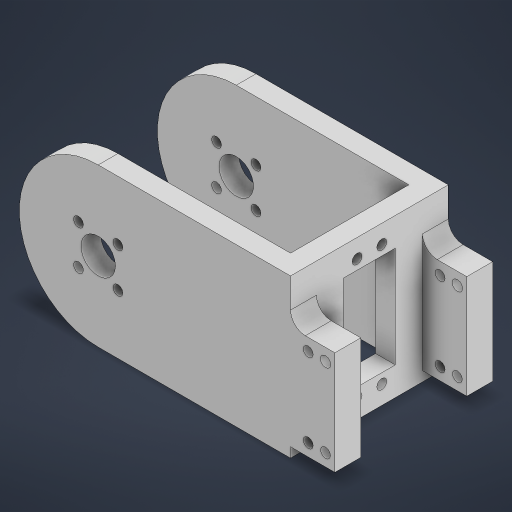
# Autodesk Inventor part: DifferentialMount
Saved by Autodesk Inventor 2024 (Build 280153000, 153)
## iProperties
Created: 2024-01-28
Part Number: DifferentialMount
Material: Generic
Document SubType Name: Modeling
Designer: avsar
Density: 1 g/cm^3
Appearance: Default
Author: avsar
Autodesk Inventor part; units mm, degrees
ref_plane "YZ Plane" through (0, 0, 0) normal (1, 0, 0) x (0, 1, 0)
ref_plane "XZ Plane" through (0, 0, 0) normal (0, 1, 0) x (-1, 0, 0)
ref_plane "XY Plane" through (0, 0, 0) normal (0, 0, 1) x (1, 0, 0)
sketch "Sketch1" plane through (0, 0, 0) normal (1, 0, 0) x (0, 1, 0)
  line L0 (-32, 32) -> (32, 32)
  line L1 (32, 32) -> (32, -32)
  line L2 (32, -32) -> (-32, -32)
  line L3 (-32, -32) -> (-32, 32)
  line L4 (-32, 32) -> (32, -32) construction
  line L5 (32, 32) -> (-32, -32) construction
  point P0 (0, 0)
  dimension "d0" = 64
  dimension "d1" = 64
  constraints: 12 end point, 2 midpoint, 2 parallel, 1 horizontal, 1 perpendicular
  measures "d0" distance of L1.end L2.end
  measures "d1" distance of L0.end L1.end
extrude "Extrusion1" add sketch "Sketch1" along normal blind 8
sketch "Sketch2" plane through (0, 0, 0) normal (-1, 0, 0) x (0, 0, 1)
  line L0 (-32, -32) -> (-24, -32)
  line L1 (-24, -32) -> (-24, 32)
  line L2 (-24, 32) -> (-32, 32)
  line L3 (-32, 32) -> (-32, -32)
  line L4 (-32, -32) -> (-24, 32) construction
  line L5 (-24, -32) -> (-32, 32) construction
  line L6 (-32, -32) -> (-32, 32) projected
  line L7 (-32, 32) -> (32, 32) projected
  line L8 (0, 32) -> (0, -32) construction
  line L9 (32, -32) -> (-32, -32) projected
  line L10 (32, -32) -> (24, -32)
  line L11 (24, -32) -> (24, 32)
  line L12 (24, 32) -> (32, 32)
  line L13 (32, 32) -> (32, -32)
  line L14 (32, -32) -> (24, 32) construction
  line L15 (24, -32) -> (32, 32) construction
  point P0 (0, 0)
  point P1 (-28, 0)
  point P2 (-32, 0)
  point P3 (28, 0)
  point P4 (32, 0)
  dimension "d4" = 8
  dimension "d5" = 64
  constraints: 26 end point, 6 midpoint, 6 symmetric about line, 2 parallel, 1 horizontal, 1 horizontal alignment, 1 perpendicular
  measures "d4" distance of L2.end L1.end
  measures "d5" distance of L1.end L0.end
extrude "Extrusion2" add sketch "Sketch2" along normal blind 102 contours L3 L2 L1 L0 | L11 L7 L13 L9
fillet "Fillet1" radius 32 4 edges at (-102, 32, -28) (-102, 32, 28) (-102, -32, 28) (-102, -32, -28)
sketch "Sketch3" plane through (0, -32, 32) normal (0, 0, 1) x (1, 0, 0)
  arc A0 (-70, 64) -> (-70, 0) centre (-70, 32) ccw construction
  circle A1 centre (-70, 32) radius 7
  circle A2 centre (-78, 40) radius 2
  circle A3 centre (-78, 24) radius 2
  circle A4 centre (-62, 24) radius 2
  circle A5 centre (-62, 40) radius 2
  point P0 (0, 32)
  point P1 (-64, 48)
  dimension "d9" = 14
  dimension "d10" = 4
  dimension "d11" = 8
  dimension "d12" = 8
  dimension "d15" = 360
  constraints: 5 centre point, 1 coincident, 9 other
  measures "d9" diameter of A1
  measures "d10" diameter of A2
  measures "d11" horizontal distance of A2.centre A0.centre
  measures "d12" horizontal distance of A0.centre A2.centre
extrude "Extrusion3" cut sketch "Sketch3" against normal through all
sketch "Sketch5" plane through (8, 0, 0) normal (1, 0, 0) x (0, 0, -1)
  circle A0 centre (-5, 24.5) radius 2
  line L0 (0, 7) -> (0, 0) construction
  circle A1 centre (5, 24.5) radius 2
  circle A2 centre (-5, -24.5) radius 2
  circle A3 centre (5, -24.5) radius 2
  line L1 (-32, 32) -> (-32, -32) construction
  line L2 (-32, 0) -> (32, 0) construction
  line L3 (32, 32) -> (32, -32) construction
  dimension "d22" = 4
  dimension "d23" = 5
  dimension "d24" = 24.5
  constraints: 4 centre point, 4 end point, 2 midpoint, 1 symmetric about line, 1 vertical, 3 other
  measures "d22" diameter of A0
  measures "d23" horizontal distance of point (0, 0) A0.centre
  measures "d24" vertical distance of point (0, 0) A0.centre
extrude "Extrusion5" cut sketch "Sketch5" against normal through all
sketch "Sketch7" plane through (8, 0, 0) normal (1, 0, 0) x (0, 0, -1)
  line L0 (-10.5, -20.5) -> (10.5, -20.5)
  line L1 (10.5, -20.5) -> (10.5, 20.5)
  line L2 (10.5, 20.5) -> (-10.5, 20.5)
  line L3 (-10.5, 20.5) -> (-10.5, -20.5)
  line L4 (-10.5, -20.5) -> (10.5, 20.5) construction
  line L5 (10.5, -20.5) -> (-10.5, 20.5) construction
  point P0 (0, 0)
  dimension "d30" = 21
  dimension "d31" = 41
  constraints: 12 end point, 2 midpoint, 2 parallel, 1 horizontal, 1 perpendicular
  measures "d30" distance of L2.end L1.end
  measures "d31" distance of L1.end L0.end
extrude "Extrusion7" cut sketch "Sketch7" against normal up to surface (8 mm away)
sketch "Sketch8" plane through (8, 0, 0) normal (1, 0, 0) x (0, 0, -1)
  line L0 (-32, -28) -> (-21.5, -28)
  line L1 (-21.5, -28) -> (-21.5, 14)
  line L2 (-21.5, 14) -> (-32, 14)
  line L3 (-32, 14) -> (-32, -28)
  line L4 (-32, -28) -> (-21.5, 14) construction
  line L5 (-21.5, -28) -> (-32, 14) construction
  line L6 (-32, 32) -> (-32, -32) construction
  line L7 (10.5, 20.5) -> (-10.5, 20.5) construction
  line L8 (0, 20.5) -> (0, -20.5) construction
  line L9 (-10.5, -20.5) -> (10.5, -20.5) construction
  line L10 (32, -28) -> (21.5, -28)
  line L11 (21.5, -28) -> (21.5, 14)
  line L12 (21.5, 14) -> (32, 14)
  line L13 (32, 14) -> (32, -28)
  line L14 (32, -28) -> (21.5, 14) construction
  line L15 (21.5, -28) -> (32, 14) construction
  point P0 (0, 0)
  point P1 (-32, 0)
  point P2 (-21.5, -7)
  point P3 (-32, 0)
  point P4 (26.75, 0)
  point P5 (32, 0)
  point P6 (21.5, -7)
  point P7 (32, 0)
  point P8 (0, 0)
  dimension "d35" = 42
  dimension "d44" = 10.5
  dimension "d45" = 7
  constraints: 22 end point, 7 symmetric about line, 6 midpoint, 2 parallel, 2 point on line, 1 horizontal, 1 perpendicular, 6 other
  measures "d35" distance of L1.end L0.end
  measures "d44" distance between parallel lines of L3 L1
  measures "d45" vertical distance of point (0, 0) point (-21.5, -7)
extrude "Extrusion8" add sketch "Sketch8" along normal blind 18
sketch "Sketch9" plane through (0, -32, 32) normal (0, 0, 1) x (1, 0, 0)
  circle A0 centre (15.2, 41) radius 2
  line L0 (8, 64) -> (8, 46) construction
  line L1 (26, 46) -> (26, 4) construction
  line L2 (26, 25) -> (0, 25) construction
  line L3 (0, 0) -> (0, 64) construction
  circle A1 centre (15.2, 9) radius 2
  point P0 (0, 32)
  dimension "d39" = 4
  dimension "d40" = 7.2
  dimension "d46" = 16
  constraints: 2 centre point, 2 end point, 1 horizontal, 1 midpoint, 1 point on line, 1 symmetric about line, 1 other
  measures "d39" diameter of A0
  measures "d40" distance from line of L0 A0.centre
  measures "d46" vertical distance of A0.centre L2.start
extrude "Extrusion9" cut sketch "Sketch9" against normal up to surface (64 mm away)
fillet "Fillet2" radius 6 2 edges at (8, 14, 26.75) (8, 14, -26.75)
sketch "Sketch10" plane through (0, -32, 32) normal (0, 0, 1) x (1, 0, 0)
  circle A0 centre (15.2, 41) radius 2 construction
  circle A1 centre (15.2, 9) radius 2 construction
  circle A2 centre (22.2, 41) radius 2.1
  circle A3 centre (22.2, 9) radius 2
  point P0 (0, 32)
  dimension "d48" = 4.2
  dimension "d49" = 7
  dimension "d50" = 4
  constraints: 2 centre point, 2 horizontal alignment, 1 vertical alignment
  measures "d48" diameter of A2
  measures "d49" distance of A2.centre A0.centre
  measures "d50" diameter of A3
extrude "Extrusion10" cut sketch "Sketch10" against normal up to surface (64 mm away)
body "Solid1"
